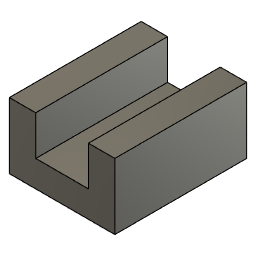
Test Bench Assembly v2 (Autodesk Fusion 360 archive; units mm, degrees)
design "Connerctor"
Autodesk Fusion 360 part; units mm, degrees
sketch "Sketch1" plane through (0, 0, 0) normal (0, 1, 0) x (1, 0, 0)
  line L0 (0, 0) -> (8, 0)
  line L1 (8, 0) -> (8, 10)
  line L2 (8, 10) -> (0, 10)
  line L3 (0, 10) -> (0, 0)
  dimension "d1" = 8
  dimension "d2" = 10
  constraint horizontal L0
  constraint vertical L1
  constraint horizontal L2
  constraint vertical L3
  constraint coincident L0.start L3.end
  measures "d1" distance of L0.start L0.end
  measures "d2" distance of L0.start L2.end
extrude "Extrude1" add sketch "Sketch1" along normal blind 2
sketch "Sketch3" plane through (0, 2, 0) normal (0, 1, 0) x (-1, 0, 0)
  line L0 (0, -10) -> (0, 0)
  line L1 (0, 0) -> (-8, 0)
  line L2 (-8, 0) -> (-8, -10)
  line L3 (-8, -10) -> (0, -10)
  line L4 (0, 0) -> (-2, 0)
  line L5 (-2, 0) -> (-2, -10)
  line L6 (-2, -10) -> (0, -10)
  line L7 (0, -10) -> (0, 0)
  line L8 (-8, 0) -> (-6, 0)
  line L9 (-6, 0) -> (-6, -10)
  line L10 (-6, -10) -> (-8, -10)
  line L11 (-8, -10) -> (-8, 0)
  dimension "d5" = 2
  dimension "d6" = 2
  constraint horizontal L4
  constraint vertical L5
  constraint horizontal L6
  constraint vertical L7
  constraint coincident L3 L5.end
  constraint coincident L0.end L1.start
  constraint horizontal L8
  constraint vertical L9
  constraint horizontal L10
  constraint vertical L11
  constraint coincident L3 L9.end
  constraint coincident L1.end L2.start
  measures "d5" distance of L0.end L4.end
  measures "d6" distance of L1.end L8.end
extrude "Extrude2" add sketch "Sketch3" along normal blind 3 contours L0 L1 L3 L4 L5 L6 L7 | L1 L2 L3 L8 L9 L10 L11

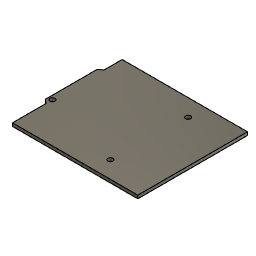
design "Nucleo-L476RG Board"
Autodesk Fusion 360 part; units mm, degrees
sketch "Sketch1" plane through (0, 0, 0) normal (0, 1, 0) x (1, 0, 0)
  line L0 (0, 0) -> (82.5, 0)
  line L1 (82.5, 0) -> (82.5, -70)
  line L2 (82.5, -70) -> (0, -70)
  line L3 (0, -70) -> (0, 0)
  line L4 (2.54, -70) -> (2.54, -48.5)
  line L5 (2.54, -48.5) -> (0, -46.5)
  line L6 (2.54, 0) -> (2.54, -11.5)
  line L7 (2.54, -11.5) -> (0, -13.5)
  dimension "d1" = 82.5
  dimension "d2" = 70
  dimension "d3" = 33
  dimension "d4" = 11.5
  dimension "d5" = 2.54
  dimension "d6" = 2.54
  dimension "d7" = 21.5
  dimension "d8" = 2
  constraint horizontal L0
  constraint vertical L1
  constraint horizontal L2
  constraint vertical L3
  constraint coincident L0.start L3.end
  constraint coincident L2 L4.start
  constraint perpendicular L2 L4
  constraint coincident L3 L5.end
  constraint coincident L0 L6.start
  constraint perpendicular L0 L6
  constraint coincident L3 L7.end
  measures "d1" distance of L1.end L2.end
  measures "d2" distance of L0.start L2.end
  measures "d3" distance of L5.end L7.end
  measures "d4" distance of L6.start L6.end
  measures "d5" distance of L3 L4
  measures "d6" distance of L3 L6
  measures "d7" distance of L4.start L4.end
  measures "d8" vertical distance of L4.end L5.end
extrude "Extrude1" add sketch "Sketch1" along normal blind 2 contours L0 L1 L2 L3 L4 L5 L6 L7
sketch "Sketch2" plane through (0, 2, 0) normal (0, 1, 0) x (-1, 0, 0)
  line L0 (-2.54, 0) -> (-2.54, 11.5)
  line L1 (-2.54, 11.5) -> (0, 13.5)
  line L2 (0, 13.5) -> (0, 46.5)
  line L3 (0, 46.5) -> (-2.54, 48.5)
  line L4 (-2.54, 48.5) -> (-2.54, 70)
  line L5 (-2.54, 70) -> (-82.5, 70)
  line L6 (-82.5, 70) -> (-82.5, 0)
  line L7 (-82.5, 0) -> (-2.54, 0)
  circle A0 centre (-2.54, 44.5) radius 1.6
  circle A1 centre (-54.14, 59.13) radius 1.6
  circle A2 centre (-55.54, 10.87) radius 1.6
  dimension "d11" = 3.2
  dimension "d12" = 2.54
  dimension "d13" = 33
  dimension "d14" = 3.2
  dimension "d15" = 3.2
  dimension "d17" = 10.87
  dimension "d20" = 53
  dimension "d21" = 51.6
  dimension "d22" = 48.26
  measures "d11" diameter of A0
  measures "d12" distance of L2 A0.centre
  measures "d13" distance of L0.end A0.centre
  measures "d14" diameter of A2
  measures "d15" diameter of A1
  measures "d17" distance of L7 A2.centre
  measures "d20" distance of L0 A2.centre
  measures "d21" distance of L4 A1.centre
  measures "d22" vertical distance of A1.centre A2.centre
extrude "Extrude2" cut sketch "Sketch2" against normal blind 2 contours A0 | A1 | A2

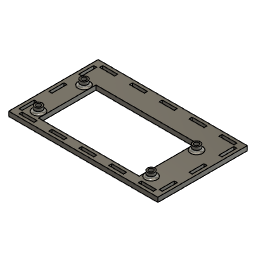
design "Modular Test Bench - LCD"
Autodesk Fusion 360 part; units mm, degrees
sketch "Sketch1" plane through (0, 0, 0) normal (0, 1, 0) x (1, 0, 0)
  line L0 (0, 0) -> (100, 0)
  line L1 (100, 0) -> (100, 60)
  line L2 (100, 60) -> (0, 60)
  line L3 (0, 60) -> (0, 0)
  dimension "d1" = 100
  dimension "d2" = 60
  constraint horizontal L0
  constraint vertical L1
  constraint horizontal L2
  constraint vertical L3
  constraint coincident L0.start L3.end
  measures "d1" distance of L0.start L0.end
  measures "d2" distance of L0.start L2.end
extrude "Extrude1" add sketch "Sketch1" along normal blind 3
sketch "Sketch2" plane through (0, 3, 0) normal (0, 1, 0) x (-1, 0, 0)
  line L0 (0, -60) -> (0, 0)
  line L1 (0, 0) -> (-100, 0)
  line L2 (-100, 0) -> (-100, -60)
  line L3 (-100, -60) -> (0, -60)
  line L4 (-5, -2) -> (-15, -2)
  line L5 (-15, -2) -> (-15, -4)
  line L6 (-15, -4) -> (-5, -4)
  line L7 (-5, -4) -> (-5, -2)
  line L8 (-25, -2) -> (-35, -2)
  line L9 (-35, -2) -> (-35, -4)
  line L10 (-35, -4) -> (-25, -4)
  line L11 (-25, -4) -> (-25, -2)
  line L12 (-45, -2) -> (-55, -2)
  line L13 (-55, -2) -> (-55, -4)
  line L14 (-55, -4) -> (-45, -4)
  line L15 (-45, -4) -> (-45, -2)
  line L16 (-65, -2) -> (-75, -2)
  line L17 (-75, -2) -> (-75, -4)
  line L18 (-75, -4) -> (-65, -4)
  line L19 (-65, -4) -> (-65, -2)
  line L20 (-5, -56) -> (-15, -56)
  line L21 (-15, -56) -> (-15, -58)
  line L22 (-15, -58) -> (-5, -58)
  line L23 (-5, -58) -> (-5, -56)
  line L24 (-25, -56) -> (-35, -56)
  line L25 (-35, -56) -> (-35, -58)
  line L26 (-35, -58) -> (-25, -58)
  line L27 (-25, -58) -> (-25, -56)
  line L28 (-45, -56) -> (-55, -56)
  line L29 (-55, -56) -> (-55, -58)
  line L30 (-55, -58) -> (-45, -58)
  line L31 (-45, -58) -> (-45, -56)
  line L32 (-65, -56) -> (-75, -56)
  line L33 (-75, -56) -> (-75, -58)
  line L34 (-75, -58) -> (-65, -58)
  line L35 (-65, -58) -> (-65, -56)
  line L36 (-4, -5) -> (-2, -5)
  line L37 (-2, -5) -> (-2, -15)
  line L38 (-2, -15) -> (-4, -15)
  line L39 (-4, -15) -> (-4, -5)
  line L40 (-98, -15) -> (-98, -5)
  line L41 (-98, -5) -> (-96, -5)
  line L42 (-96, -5) -> (-96, -15)
  line L43 (-96, -15) -> (-98, -15)
  line L44 (-4, -35) -> (-4, -25)
  line L45 (-4, -25) -> (-2, -25)
  line L46 (-2, -25) -> (-2, -35)
  line L47 (-2, -35) -> (-4, -35)
  line L48 (-98, -35) -> (-98, -25)
  line L49 (-98, -25) -> (-96, -25)
  line L50 (-96, -25) -> (-96, -35)
  line L51 (-96, -35) -> (-98, -35)
  line L52 (-85, -2) -> (-95, -2)
  line L53 (-95, -2) -> (-95, -4)
  line L54 (-95, -4) -> (-85, -4)
  line L55 (-85, -4) -> (-85, -2)
  line L56 (-85, -56) -> (-95, -56)
  line L57 (-95, -56) -> (-95, -58)
  line L58 (-95, -58) -> (-85, -58)
  line L59 (-85, -58) -> (-85, -56)
  line L60 (-4, -55) -> (-4, -45)
  line L61 (-4, -45) -> (-2, -45)
  line L62 (-2, -45) -> (-2, -55)
  line L63 (-2, -55) -> (-4, -55)
  line L64 (-98, -55) -> (-98, -45)
  line L65 (-98, -45) -> (-96, -45)
  line L66 (-96, -45) -> (-96, -55)
  line L67 (-96, -55) -> (-98, -55)
  dimension "d5" = 2
  dimension "d6" = 5
  dimension "d7" = 10
  dimension "d8" = 2
  dimension "d11" = -20
  dimension "d12" = -54
  dimension "d13" = 2
  dimension "d14" = 2
  dimension "d15" = 5
  dimension "d16" = 10
  dimension "d19" = -94
  dimension "d20" = -20
  constraint horizontal L4
  constraint vertical L5
  constraint horizontal L6
  constraint vertical L7
  constraint horizontal L36
  constraint vertical L37
  constraint horizontal L38
  constraint vertical L39
  measures "d5" distance of L1 L4
  measures "d6" distance of L0 L7
  measures "d7" distance of L4.start L4.end
  measures "d8" distance of L4.start L6.end
  measures "d13" distance of L36.start L36.end
  measures "d14" distance of L0 L37
  measures "d15" distance of L1 L36
  measures "d16" distance of L36.start L38.end
extrude "Extrude2" cut sketch "Sketch2" against normal blind 3 contours L4 L5 L6 L7 | L8 L9 L10 L11 | L12 L13 L14 L15 | L16 L17 L18 L19 | L20 L21 L22 L23 | L24 L25 L26 L27 | L28 L29 L30 L31 | L32 L33 L34 L35 | L36 L37 L38 L39 | L40 L41 L42 L43 | L44 L45 L46 L47 | L48 L49 L50 L51 | L52 L53 L54 L55 | L56 L57 L58 L59 | L60 L61 L62 L63 | L64 L65 L66 L67
sketch "Sketch3" plane through (0, 3, 0) normal (0, 1, 0) x (-1, 0, 0)
  line L0 (-4, -25) -> (-2, -25)
  line L1 (-2, -25) -> (-2, -35)
  line L2 (-2, -35) -> (-4, -35)
  line L3 (-4, -35) -> (-4, -25)
  line L4 (-75, -2) -> (-65, -2)
  line L5 (-65, -2) -> (-65, -4)
  line L6 (-65, -4) -> (-75, -4)
  line L7 (-75, -4) -> (-75, -2)
  line L8 (-55, -2) -> (-45, -2)
  line L9 (-45, -2) -> (-45, -4)
  line L10 (-45, -4) -> (-55, -4)
  line L11 (-55, -4) -> (-55, -2)
  line L12 (-2, -5) -> (-2, -15)
  line L13 (-2, -15) -> (-4, -15)
  line L14 (-4, -15) -> (-4, -5)
  line L15 (-4, -5) -> (-2, -5)
  line L16 (-15, -56) -> (-5, -56)
  line L17 (-5, -56) -> (-5, -58)
  line L18 (-5, -58) -> (-15, -58)
  line L19 (-15, -58) -> (-15, -56)
  line L20 (-55, -56) -> (-45, -56)
  line L21 (-45, -56) -> (-45, -58)
  line L22 (-45, -58) -> (-55, -58)
  line L23 (-55, -58) -> (-55, -56)
  line L24 (-75, -56) -> (-65, -56)
  line L25 (-65, -56) -> (-65, -58)
  line L26 (-65, -58) -> (-75, -58)
  line L27 (-75, -58) -> (-75, -56)
  line L28 (-15, -2) -> (-5, -2)
  line L29 (-5, -2) -> (-5, -4)
  line L30 (-5, -4) -> (-15, -4)
  line L31 (-15, -4) -> (-15, -2)
  line L32 (-35, -56) -> (-25, -56)
  line L33 (-25, -56) -> (-25, -58)
  line L34 (-25, -58) -> (-35, -58)
  line L35 (-35, -58) -> (-35, -56)
  line L36 (-98, -25) -> (-96, -25)
  line L37 (-96, -25) -> (-96, -35)
  line L38 (-96, -35) -> (-98, -35)
  line L39 (-98, -35) -> (-98, -25)
  line L40 (-35, -2) -> (-25, -2)
  line L41 (-25, -2) -> (-25, -4)
  line L42 (-25, -4) -> (-35, -4)
  line L43 (-35, -4) -> (-35, -2)
  line L44 (-98, -5) -> (-96, -5)
  line L45 (-96, -5) -> (-96, -15)
  line L46 (-96, -15) -> (-98, -15)
  line L47 (-98, -15) -> (-98, -5)
  line L48 (0, -60) -> (0, 0)
  line L49 (0, 0) -> (-100, 0)
  line L50 (-100, 0) -> (-100, -60)
  line L51 (-100, -60) -> (0, -60)
  circle A0 centre (-10, -10) radius 1.5
  circle A1 centre (-85.5, -10) radius 1.5
  line L52 (-95, -56) -> (-85, -56)
  line L53 (-85, -56) -> (-85, -58)
  line L54 (-85, -58) -> (-95, -58)
  line L55 (-95, -58) -> (-95, -56)
  line L56 (-95, -2) -> (-85, -2)
  line L57 (-85, -2) -> (-85, -4)
  line L58 (-85, -4) -> (-95, -4)
  line L59 (-95, -4) -> (-95, -2)
  circle A2 centre (-10, -40.5) radius 1.5
  circle A3 centre (-85.5, -40.5) radius 1.5
  line L60 (-4, -45) -> (-2, -45)
  line L61 (-2, -45) -> (-2, -55)
  line L62 (-2, -55) -> (-4, -55)
  line L63 (-4, -55) -> (-4, -45)
  line L64 (-98, -45) -> (-96, -45)
  line L65 (-96, -45) -> (-96, -55)
  line L66 (-96, -55) -> (-98, -55)
  line L67 (-98, -55) -> (-98, -45)
  dimension "d23" = 75.5
  dimension "d24" = 30.5
  dimension "d25" = 10
  dimension "d26" = 10
  dimension "d27" = 3
  dimension "d28" = 3
  dimension "d29" = 3
  dimension "d30" = 3
  constraint vertical A0.centre A2.centre
  constraint horizontal A0.centre A1.centre
  constraint horizontal A2.centre A3.centre
  constraint vertical A1.centre A3.centre
  measures "d23" horizontal distance of A0.centre A1.centre
  measures "d24" distance of A0.centre A2.centre
  measures "d25" distance of L49 A0.centre
  measures "d26" distance of L48 A0.centre
  measures "d27" diameter of A0
  measures "d28" diameter of A1
  measures "d29" diameter of A2
  measures "d30" diameter of A3
extrude "Extrude3" cut sketch "Sketch3" against normal blind 3 contours A0 | A1 | A2 | A3
sketch "Sketch4" plane through (0, 3, 0) normal (0, 1, 0) x (-1, 0, 0)
  circle A0 centre (-10, -40.5) radius 1.5
  circle A1 centre (-85.5, -40.5) radius 1.5
  circle A2 centre (-10, -10) radius 1.5
  circle A3 centre (-85.5, -10) radius 1.5
  line L0 (-95, -2) -> (-85, -2)
  line L1 (-85, -2) -> (-85, -4)
  line L2 (-85, -4) -> (-95, -4)
  line L3 (-95, -4) -> (-95, -2)
  line L4 (-4, -25) -> (-2, -25)
  line L5 (-2, -25) -> (-2, -35)
  line L6 (-2, -35) -> (-4, -35)
  line L7 (-4, -35) -> (-4, -25)
  line L8 (-75, -2) -> (-65, -2)
  line L9 (-65, -2) -> (-65, -4)
  line L10 (-65, -4) -> (-75, -4)
  line L11 (-75, -4) -> (-75, -2)
  line L12 (-55, -2) -> (-45, -2)
  line L13 (-45, -2) -> (-45, -4)
  line L14 (-45, -4) -> (-55, -4)
  line L15 (-55, -4) -> (-55, -2)
  line L16 (-2, -5) -> (-2, -15)
  line L17 (-2, -15) -> (-4, -15)
  line L18 (-4, -15) -> (-4, -5)
  line L19 (-4, -5) -> (-2, -5)
  line L20 (-15, -56) -> (-5, -56)
  line L21 (-5, -56) -> (-5, -58)
  line L22 (-5, -58) -> (-15, -58)
  line L23 (-15, -58) -> (-15, -56)
  line L24 (-55, -56) -> (-45, -56)
  line L25 (-45, -56) -> (-45, -58)
  line L26 (-45, -58) -> (-55, -58)
  line L27 (-55, -58) -> (-55, -56)
  line L28 (-4, -45) -> (-2, -45)
  line L29 (-2, -45) -> (-2, -55)
  line L30 (-2, -55) -> (-4, -55)
  line L31 (-4, -55) -> (-4, -45)
  line L32 (-95, -56) -> (-85, -56)
  line L33 (-85, -56) -> (-85, -58)
  line L34 (-85, -58) -> (-95, -58)
  line L35 (-95, -58) -> (-95, -56)
  line L36 (-75, -56) -> (-65, -56)
  line L37 (-65, -56) -> (-65, -58)
  line L38 (-65, -58) -> (-75, -58)
  line L39 (-75, -58) -> (-75, -56)
  line L40 (-15, -2) -> (-5, -2)
  line L41 (-5, -2) -> (-5, -4)
  line L42 (-5, -4) -> (-15, -4)
  line L43 (-15, -4) -> (-15, -2)
  line L44 (-35, -56) -> (-25, -56)
  line L45 (-25, -56) -> (-25, -58)
  line L46 (-25, -58) -> (-35, -58)
  line L47 (-35, -58) -> (-35, -56)
  line L48 (-98, -25) -> (-96, -25)
  line L49 (-96, -25) -> (-96, -35)
  line L50 (-96, -35) -> (-98, -35)
  line L51 (-98, -35) -> (-98, -25)
  line L52 (-35, -2) -> (-25, -2)
  line L53 (-25, -2) -> (-25, -4)
  line L54 (-25, -4) -> (-35, -4)
  line L55 (-35, -4) -> (-35, -2)
  line L56 (-98, -5) -> (-96, -5)
  line L57 (-96, -5) -> (-96, -15)
  line L58 (-96, -15) -> (-98, -15)
  line L59 (-98, -15) -> (-98, -5)
  line L60 (-98, -45) -> (-96, -45)
  line L61 (-96, -45) -> (-96, -55)
  line L62 (-96, -55) -> (-98, -55)
  line L63 (-98, -55) -> (-98, -45)
  line L64 (0, -60) -> (0, 0)
  line L65 (0, 0) -> (-100, 0)
  line L66 (-100, 0) -> (-100, -60)
  line L67 (-100, -60) -> (0, -60)
  circle A4 centre (-10, -10) radius 2.5
  circle A5 centre (-10, -40.5) radius 2.5
  circle A6 centre (-85.5, -40.5) radius 2.5
  circle A7 centre (-85.5, -10) radius 2.5
  dimension "d33" = 5
  dimension "d34" = 5
  dimension "d35" = 5
  dimension "d36" = 5
  constraint concentric A2 A4
  constraint concentric A0 A5
  constraint concentric A1 A6
  constraint concentric A3 A7
  measures "d33" diameter of A7
  measures "d34" diameter of A6
  measures "d35" diameter of A5
  measures "d36" diameter of A4
extrude "Extrude4" add sketch "Sketch4" along normal blind 3.5 contours A4 | A5 | A6 | A7
sketch "Sketch5" plane through (0, 3, 0) normal (0, 1, 0) x (-1, 0, 0)
  circle A0 centre (-85.5, -10) radius 2.5
  circle A1 centre (-10, -40.5) radius 2.5
  circle A2 centre (-85.5, -40.5) radius 2.5
  circle A3 centre (-10, -10) radius 2.5
  line L0 (-95, -2) -> (-85, -2)
  line L1 (-85, -2) -> (-85, -4)
  line L2 (-85, -4) -> (-95, -4)
  line L3 (-95, -4) -> (-95, -2)
  line L4 (-4, -25) -> (-2, -25)
  line L5 (-2, -25) -> (-2, -35)
  line L6 (-2, -35) -> (-4, -35)
  line L7 (-4, -35) -> (-4, -25)
  line L8 (-75, -2) -> (-65, -2)
  line L9 (-65, -2) -> (-65, -4)
  line L10 (-65, -4) -> (-75, -4)
  line L11 (-75, -4) -> (-75, -2)
  line L12 (-55, -2) -> (-45, -2)
  line L13 (-45, -2) -> (-45, -4)
  line L14 (-45, -4) -> (-55, -4)
  line L15 (-55, -4) -> (-55, -2)
  line L16 (-2, -5) -> (-2, -15)
  line L17 (-2, -15) -> (-4, -15)
  line L18 (-4, -15) -> (-4, -5)
  line L19 (-4, -5) -> (-2, -5)
  line L20 (-15, -56) -> (-5, -56)
  line L21 (-5, -56) -> (-5, -58)
  line L22 (-5, -58) -> (-15, -58)
  line L23 (-15, -58) -> (-15, -56)
  line L24 (-55, -56) -> (-45, -56)
  line L25 (-45, -56) -> (-45, -58)
  line L26 (-45, -58) -> (-55, -58)
  line L27 (-55, -58) -> (-55, -56)
  line L28 (-4, -45) -> (-2, -45)
  line L29 (-2, -45) -> (-2, -55)
  line L30 (-2, -55) -> (-4, -55)
  line L31 (-4, -55) -> (-4, -45)
  line L32 (-95, -56) -> (-85, -56)
  line L33 (-85, -56) -> (-85, -58)
  line L34 (-85, -58) -> (-95, -58)
  line L35 (-95, -58) -> (-95, -56)
  line L36 (-75, -56) -> (-65, -56)
  line L37 (-65, -56) -> (-65, -58)
  line L38 (-65, -58) -> (-75, -58)
  line L39 (-75, -58) -> (-75, -56)
  line L40 (-15, -2) -> (-5, -2)
  line L41 (-5, -2) -> (-5, -4)
  line L42 (-5, -4) -> (-15, -4)
  line L43 (-15, -4) -> (-15, -2)
  line L44 (-35, -56) -> (-25, -56)
  line L45 (-25, -56) -> (-25, -58)
  line L46 (-25, -58) -> (-35, -58)
  line L47 (-35, -58) -> (-35, -56)
  line L48 (-98, -25) -> (-96, -25)
  line L49 (-96, -25) -> (-96, -35)
  line L50 (-96, -35) -> (-98, -35)
  line L51 (-98, -35) -> (-98, -25)
  line L52 (-35, -2) -> (-25, -2)
  line L53 (-25, -2) -> (-25, -4)
  line L54 (-25, -4) -> (-35, -4)
  line L55 (-35, -4) -> (-35, -2)
  line L56 (-98, -5) -> (-96, -5)
  line L57 (-96, -5) -> (-96, -15)
  line L58 (-96, -15) -> (-98, -15)
  line L59 (-98, -15) -> (-98, -5)
  line L60 (-98, -45) -> (-96, -45)
  line L61 (-96, -45) -> (-96, -55)
  line L62 (-96, -55) -> (-98, -55)
  line L63 (-98, -55) -> (-98, -45)
  line L64 (0, -60) -> (0, 0)
  line L65 (0, 0) -> (-100, 0)
  line L66 (-100, 0) -> (-100, -60)
  line L67 (-100, -60) -> (0, -60)
  line L68 (-81.5, -6) -> (-14, -6)
  line L69 (-14, -6) -> (-14, -44.5)
  line L70 (-14, -44.5) -> (-81.5, -44.5)
  line L71 (-81.5, -44.5) -> (-81.5, -6)
  dimension "d39" = 4
  dimension "d40" = 6
  dimension "d42" = 15.5
  dimension "d43" = 4
  constraint horizontal L68
  constraint vertical L69
  constraint horizontal L70
  constraint vertical L71
  measures "d39" distance of A0.centre L71
  measures "d40" distance of L65 L68
  measures "d42" distance of L67 L70
  measures "d43" distance of A3.centre L69
extrude "Extrude5" cut sketch "Sketch5" against normal blind 3 contours L68 L69 L70 L71
fillet "Fillet1" radius 1.5 4 edges at (12.3308, 3, -9.096) (12.3308, 3, -39.596) (87.8308, 3, -39.596) (87.8308, 3, -9.096)
